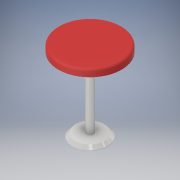
# Autodesk Inventor part: Stool
Saved by Autodesk Inventor 2017 (Build 210142000, 142)
## iProperties
Created: 2017-02-11
Part Number: Stool
Material: Aluminum 6061, Welded
Document SubType Name: Modeling
Designer: TheMasterTechnician
Density: 2.7 g/cm^3
Appearance: Weld - Aluminum
Author: TheMasterTechnician
Autodesk Inventor part; units mm, degrees
ref_plane "YZ Plane" through (0, 0, 0) normal (1, 0, 0) x (0, 1, 0)
ref_plane "XZ Plane" through (0, 0, 0) normal (0, 1, 0) x (-1, 0, 0)
ref_plane "XY Plane" through (0, 0, 0) normal (0, 0, 1) x (1, 0, 0)
sketch "Sketch1" plane through (0, 0, 0) normal (0, 1, 0) x (-1, 0, 0)
  circle A0 centre (0, 0) radius 228.6
  dimension "d0" = 457.2
  constraints: 1 centre point, 1 coincident
  measures "d0" diameter of A0
extrude "Extrusion1" add sketch "Sketch1" along normal blind 50.8
fillet "Fillet1" radius 15.85 1 edges at (228.6, 50.8, 0)
sketch "Sketch2" plane through (0, 0, 0) normal (0, -1, 0) x (1, 0, 0)
  circle A0 centre (0, 0) radius 25.4
  dimension "d4" = 50.8
  constraints: 1 centre point, 1 coincident
  measures "d4" diameter of A0
extrude "Extrusion2" add sketch "Sketch2" along normal blind 508
sketch "Sketch3" plane through (0, -508, 0) normal (0, -1, 0) x (1, 0, 0)
  circle A0 centre (0, 0) radius 127
  dimension "d7" = 254
  constraints: 1 centre point, 1 coincident
  measures "d7" diameter of A0
extrude "Extrusion3" add sketch "Sketch3" along normal blind 25.4
chamfer "Chamfer1" distance 21.8125 angle 45 1 edges at (-127, -508, 0)
body "Solid1"
